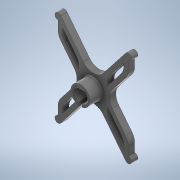
# Autodesk Inventor part: ButterflyEncoderBracket
Saved by Autodesk Inventor 2020 (Build 240168000, 168)
## iProperties
Created: 2019-06-02
Part Number: ButterflyEncoderBracket
Material: ABS Plastic
Document SubType Name: Modeling
Designer: Connor
Density: 1.06 g/cm^3
Appearance: Smooth - Black
Author: Connor
Autodesk Inventor part; units mm, degrees
ref_plane "YZ Plane" through (0, 0, 0) normal (1, 0, 0) x (0, 1, 0)
ref_plane "XZ Plane" through (0, 0, 0) normal (0, 1, 0) x (-1, 0, 0)
ref_plane "XY Plane" through (0, 0, 0) normal (0, 0, 1) x (1, 0, 0)
sketch "Sketch1" plane through (0, 0, 0) normal (0, 0, 1) x (1, 0, 0)
  line L0 (-17.4625, 22.225) -> (17.4625, 22.225) construction
  line L1 (17.4625, 22.225) -> (17.4625, -22.225) construction
  line L2 (17.4625, -22.225) -> (-17.4625, -22.225) construction
  line L3 (-17.4625, -22.225) -> (-17.4625, 22.225) construction
  line L4 (-17.4625, 22.225) -> (17.4625, -22.225) construction
  line L5 (-17.4625, -22.225) -> (17.4625, 22.225) construction
  circle A0 centre (-17.4625, 22.225) radius 1.5875
  circle A1 centre (17.4625, 22.225) radius 1.5875
  circle A2 centre (17.4625, -22.225) radius 1.5875
  circle A3 centre (-17.4625, -22.225) radius 1.5875
  circle A4 centre (0, 0) radius 6.35
  line L6 (-17.4625, 20.6375) -> (-17.4625, 14.1432)
  line L7 (-17.4625, 14.1432) -> (-6.35, 0)
  line L8 (-17.4625, 0) -> (17.4625, 0) construction
  line L9 (-15.269, 18.4523) -> (-15.269, 14.9018)
  line L10 (-15.269, 14.9018) -> (-7.1883, 4.6174)
  line L11 (-15.269, 18.4523) -> (-15.269, 22.0027) construction
  line L12 (-15.269, 14.9018) -> (-15.269, 11.3514) construction
  line L13 (0, 22.225) -> (0, -22.225) construction
  circle A5 centre (17.4625, 22.225) radius 1.5875
  line L14 (17.4625, 20.6375) -> (17.4625, 14.1432)
  line L15 (17.4625, 14.1432) -> (6.35, 0)
  line L16 (15.269, 18.4523) -> (15.269, 14.9018)
  line L17 (15.269, 14.9018) -> (7.1883, 4.6174)
  circle A6 centre (-17.4625, -22.225) radius 1.5875
  circle A7 centre (17.4625, -22.225) radius 1.5875
  line L18 (-17.4625, -20.6375) -> (-17.4625, -14.1432)
  line L19 (-17.4625, -14.1432) -> (-6.35, 0)
  line L20 (-15.269, -18.4523) -> (-15.269, -14.9018)
  line L21 (-15.269, -14.9018) -> (-7.1883, -4.6174)
  line L22 (15.269, -18.4523) -> (15.269, -14.9018)
  line L23 (15.269, -14.9018) -> (7.1883, -4.6174)
  line L24 (17.4625, -14.1432) -> (6.35, 0)
  line L25 (17.4625, -20.6375) -> (17.4625, -14.1432)
  circle A8 centre (0, 0) radius 3.175
  line L26 (-2.5503, 5.8154) -> (-16.2142, 23.2058)
  line L27 (2.5503, 5.8154) -> (16.2142, 23.2058)
  line L28 (-2.5503, -5.8154) -> (-16.2142, -23.2058)
  line L29 (2.5503, -5.8154) -> (16.2142, -23.2058)
  line L30 (-15.269, 18.4523) -> (-5.7416, 6.3266)
  line L31 (-15.269, -18.4523) -> (-5.7416, -6.3266)
  line L32 (15.269, 18.4523) -> (5.7416, 6.3266)
  line L33 (15.269, -18.4523) -> (5.7416, -6.3266)
  circle A9 centre (0, 0) radius 8.5435 construction
  arc A10 (-5.7416, 6.3266) -> (-7.1883, 4.6174) centre (0, 0) ccw
  arc A11 (7.1883, 4.6174) -> (5.7416, 6.3266) centre (0, 0) ccw
  arc A12 (-7.1883, -4.6174) -> (-5.7416, -6.3266) centre (0, 0) ccw
  arc A13 (5.7416, -6.3266) -> (7.1883, -4.6174) centre (0, 0) ccw
  line L34 (-2.1767, 2.3114) -> (2.1767, 2.3114)
  line L35 (-7.1883, 4.6174) -> (-7.1883, 8.1678)
  line L36 (7.1883, 4.6174) -> (7.1883, 8.1678)
  line L37 (-7.1883, -4.6174) -> (-7.1883, -8.1678)
  line L38 (7.1883, -4.6174) -> (7.1883, -8.1678)
  line L39 (-13.5329, 16.2428) -> (-11.8081, 17.598) construction
  line L40 (-17.4625, 19.0886) -> (-15.269, 19.0886) construction
  line L41 (-5.2784, 6.7179) -> (-3.9232, 4.9931) construction
  point P0 (-15.875, 22.225)
  point P1 (6.35, 0)
  point P2 (6.35, 0)
  point P3 (2.5503, -5.8154)
  point P4 (2.5503, 5.8154)
  point P5 (-2.5503, -5.8154)
  point P6 (-5.9495, -2.2196)
  point P7 (5.9495, -2.2196)
  point P8 (5.9495, 2.2196)
  point P9 (5.7416, 6.3266)
  point P10 (5.7416, -6.3266)
  point P11 (-5.7416, -6.3266)
  point P12 (16.2142, 23.2058)
  point P13 (16.2142, -23.2058)
  point P14 (-16.2142, -23.2058)
  point P15 (7.1883, -8.1678)
  point P16 (-7.1883, -8.1678)
  point P17 (7.1883, 8.1678)
  dimension "d0" = 34.925
  dimension "d1" = 44.45
  dimension "d2" = 3.175
  dimension "d4" = 12.7
  dimension "d10" = 6.35
  dimension "d22" = 5.4864
  constraints: 84 end point, 34 symmetric about line, 19 point on circle, 14 point on line, 12 centre point, 8 parallel, 7 coincident, 5 midpoint, 4 equal length, 3 equal radius, 3 perpendicular, 2 horizontal, 2 vertical alignment, 1 collinear, 1 tangent, 10 other
  measures "d0" distance of L1.end L2.end
  measures "d1" distance of L0.end L1.end
  measures "d2" diameter of A0
  measures "d4" diameter of A4
  measures "d10" diameter of A8
extrude "Extrusion1" add sketch "Sketch1" along normal blind 3.175 contours A0 | A0 L26 A4 L7 L6 | A4 | L27 A1 L14 L15 A4 | A4 L28 A3 L18 L19 | L24 L25 A2 L29 A4 | A1 | A3 | A2 | L30 A10 L35 | L36 A11 L32 | L37 A12 L31 | L33 A13 L38 | L34 A8 picked at (-0.114, 2.5931)
fillet "Fillet1" radius 6.35 18 edges at (-6.35, 0, 1.5875) (17.4625, -14.1432, 1.5875) (-17.4625, -14.1432, 1.5875) (-17.4625, 14.1432, 1.5875) (17.4625, 14.1432, 1.5875) (-15.269, -14.9018, 1.5875) (-15.269, 14.9018, 1.5875) (6.35, 0, 1.5875) (-2.5503, -5.8154, 1.5875) (2.5503, -5.8154, 1.5875) (-2.5503, 5.8154, 1.5875) (2.5503, 5.8154, 1.5875) (-7.1883, 8.1678, 1.5875) (7.1883, 8.1678, 1.5875) (-7.1883, -8.1678, 1.5875) (7.1883, -8.1678, 1.5875) (15.269, 14.9018, 1.5875) (15.269, -14.9018, 1.5875)
sketch "Sketch2" plane through (0, 0, 3.175) normal (0, 0, 1) x (1, 0, 0)
  circle A0 centre (0, 0) radius 4.7625
  arc A1 (-2.1767, 2.3114) -> (2.1767, 2.3114) centre (0, 0) ccw projected
  line L0 (0, 4.7625) -> (4.7625, 4.7625)
  line L1 (4.7625, 4.7625) -> (4.7625, 0)
  line L2 (-0.7937, -3.0742) -> (-0.7937, -4.6959)
  line L3 (0.7938, -4.6959) -> (0.7938, -3.0742)
  line L4 (-2.1767, 2.3114) -> (2.1767, 2.3114) projected
  dimension "d11" = 9.525
  dimension "d23" = 1.5875
  constraints: 8 end point, 6 point on circle, 2 parallel, 2 tangent, 2 vertical, 1 centre point, 1 coincident, 1 horizontal
  measures "d11" diameter of A0
  measures "d23" distance between parallel lines of L3 L2
extrude "Extrusion2" add sketch "Sketch2" along normal blind 6.35 contours A0 L3 A1 L4 L2
fillet "Fillet2" radius 0.7937 7 edges at (0, 4.7625, 3.175) (0, 2.3114, 9.525) (-3.0752, -0.7897, 9.525) (3.0752, -0.7897, 9.525) (0, -3.175, 3.175) (0, 2.3114, 0) (0, -3.175, 0)
body "Solid1"
